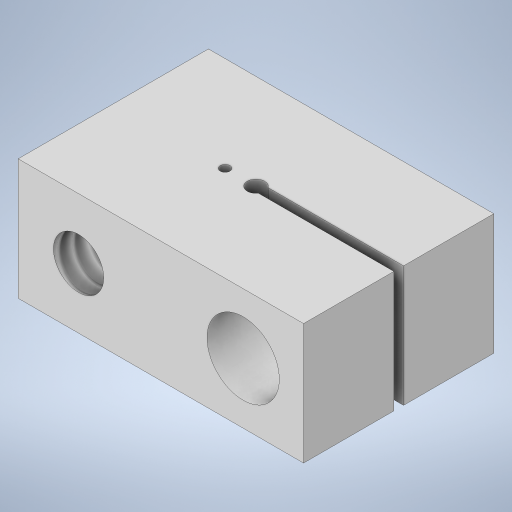
# Autodesk Inventor part: clamp(6-32)-th
Saved by Autodesk Inventor 2024 (Build 280153000, 153)
## iProperties
Created: 2023-04-27
Part Number: clamp(6-32)-th
Material: Generic
Document SubType Name: Modeling
Designer: Fujitsu
Density: 1 g/cm^3
Appearance: Default
Author: Fujitsu
Autodesk Inventor part; units mm, degrees
ref_plane "YZ Plane" through (0, 0, 0) normal (1, 0, 0) x (0, 1, 0)
ref_plane "XZ Plane" through (0, 0, 0) normal (0, 1, 0) x (-1, 0, 0)
ref_plane "XY Plane" through (0, 0, 0) normal (0, 0, 1) x (1, 0, 0)
sketch "Sketch1" plane through (0, 0, 0) normal (0, 1, 0) x (-1, 0, 0)
  line L0 (0, 0) -> (15, 0)
  line L1 (15, 0) -> (15, -10)
  line L2 (15, -10) -> (0, -10)
  line L3 (0, -10) -> (0, 0)
  line L4 (0, -5) -> (7.5006, -5)
  circle A0 centre (7.5006, -5) radius 0.4572
  line L5 (0, -5.254) -> (7.1205, -5.254)
  line L6 (0, -4.746) -> (7.1205, -4.746)
  dimension "d0" = 15
  dimension "d1" = 10
  dimension "d2" = 7.5006
  dimension "d3" = 0.9144
  dimension "d4" = 0.254
  dimension "d5" = 0.254
  constraints: 14 end point, 4 parallel, 2 horizontal, 2 point on circle, 1 centre point, 1 coincident, 1 midpoint, 1 perpendicular
  measures "d0" distance of L1.end L2.end
  measures "d1" distance of L0.end L1.end
  measures "d2" distance of L4.start L4.end
  measures "d3" diameter of A0
  measures "d4" distance between parallel lines of L4 L5
  measures "d5" distance between parallel lines of L4 L6
extrude "Extrusion1" add sketch "Sketch1" along normal blind 6.35 contours L0 L1 L2 L3 L5 A0 L6
sketch "Sketch2" plane through (-15, 0, 0) normal (0, 0, 1) x (1, 0, 0)
  line L0 (7.8795, 0) -> (15, 0) projected
  line L1 (15, 0) -> (8.65, 6.35)
  line L2 (15, 6.35) -> (7.8795, 6.35) projected
  line L3 (15, 0) -> (23.9803, 0) construction
  circle A0 centre (11.825, 3.175) radius 1.7526
  line L4 (15, 0) -> (0, 0) projected
  line L5 (0, 0) -> (6.35, 6.35)
  line L6 (7.0422, 6.35) -> (7.8795, 6.35) projected
  line L7 (0, 0) -> (8.9803, 0) construction
  circle A1 centre (3.175, 3.175) radius 1.7526
  dimension "d8" = 135
  dimension "d9" = 3.5052
  dimension "d10" = 45
  dimension "d11" = 3.5052
  constraints: 8 end point, 2 centre point, 2 equal length, 2 horizontal, 2 midpoint, 2 point on line
  measures "d8" angle of L3 L1
  measures "d9" diameter of A0
  measures "d10" angle of L7 L5
  measures "d11" diameter of A1
sketch "Sketch3" plane through (-15, 0, -10) normal (-1, 0, 0) x (0, 0, 1)
  line L0 (0, 6.35) -> (10, 6.35) projected
  line L1 (0, 6.35) -> (10, 0)
  circle A0 centre (5, 3.175) radius 0.508
  dimension "d30" = 1.016
  constraints: 2 end point, 1 centre point, 1 midpoint
  measures "d30" diameter of A0
extrude "Extrusion2" cut sketch "Sketch3" against normal blind 3.5001
hole "Hole3" at (-11.825, 3.175, 0) direction (0, 0, -1) diameter 2.6416 end through all thread size "6-32 UNC" class "2B" standard "ANSI Unified Screw Threads"
sketch "Sketch4" plane through (0, 0, -10) normal (0, 0, -1) x (-1, 0, 0)
  line L0 (0, 0) -> (6.35, 6.35)
  line L1 (7.1205, 6.35) -> (0, 6.35) projected
  line L2 (0, 0) -> (8.9803, 0) construction
  line L3 (6.35, 6.35) -> (3.175, 3.175)
  circle A0 centre (3.175, 3.175) radius 1.3208
  dimension "d44" = 45
  dimension "d45" = 2.6416
  constraints: 6 end point, 1 centre point, 1 coincident, 1 equal length, 1 horizontal, 1 midpoint, 1 point on line
  measures "d44" angle of L2 L0
  measures "d45" diameter of A0
hole "Hole4" at (-3.175, 3.175, -10) direction (0, 0, 1) diameter 2.6416 depth 5 tip angle 118 thread size "6-32 UNC" class "2B" standard "ANSI Unified Screw Threads"
hole "Hole5" at (-3.175, 3.175, 0) direction (0, 0, -1) diameter 3.7973 depth 5 tip angle 118 clearance for "Flat Head Machine Screw (82)" size "#6" standard "Ansi Unified Screw Threads"
sketch "Sketch5" plane through (0, 6.35, 0) normal (0, 1, 0) x (1, 0, 0)
  arc A0 (-7.1205, 5.254) -> (-7.1205, 4.746) centre (-7.5006, 5) ccw projected
  circle A1 centre (-7.5006, 5) radius 3.81
  circle A2 centre (-7.5006, 5) radius 16.51
  line L0 (-15, 10) -> (-15, 0) projected
  line L1 (-15, 0) -> (-8.65, 0)
  line L2 (-8.65, 0) -> (-8.65, -6.35)
  line L3 (-8.65, -6.35) -> (-15, -6.35)
  line L4 (-15, -6.35) -> (-15, 0)
  line L5 (-15, 10) -> (-8.65, 10)
  line L6 (-8.65, 10) -> (-8.65, 16.35)
  line L7 (-8.65, 16.35) -> (-15, 16.35)
  line L8 (-15, 16.35) -> (-15, 10)
  circle A3 centre (-7.5006, 5) radius 18.4277
  line L9 (-11.825, -9.8552) -> (-14.6952, -9.8552)
  line L10 (-14.6952, -9.8552) -> (-14.6952, -6.35)
  line L11 (-11.825, -9.8552) -> (-8.9548, -9.8552)
  line L12 (-8.9548, -9.8552) -> (-8.9548, -6.35)
  point P0 (0, 0)
  dimension "d60" = 7.62
  dimension "d61" = 33.02
  dimension "d62" = 6.35
  dimension "d63" = 6.35
  dimension "d64" = 6.35
  dimension "d65" = 6.35
  dimension "d66" = 36.8554
  dimension "d68" = 2.8702
  dimension "d69" = 2.8702
  constraints: 24 end point, 4 parallel, 4 perpendicular, 3 centre point, 3 coincident, 2 horizontal, 2 point on line, 1 vertical
  measures "d60" diameter of A1
  measures "d61" diameter of A2
  measures "d62" distance of L2.end L3.end
  measures "d63" distance of L1.end L2.end
  measures "d64" distance of L7.end L6.end
  measures "d65" distance of L6.end L5.end
  measures "d66" diameter of A3
  measures "d68" distance of L9.start L9.end
  measures "d69" distance of L9.start L11.end
sketch "Sketch6" plane through (0, 6.35, 0) normal (0, 1, 0) x (1, 0, 0)
  arc A0 (-7.1205, 5.254) -> (-7.1205, 4.746) centre (-7.5006, 5) ccw projected
  line L0 (-7.9578, 5) -> (-8.8722, 5)
  line L1 (-8.8722, 5) -> (-9.3802, 5)
  circle A1 centre (-9.1262, 5) radius 0.254
  point P0 (0, 0)
  dimension "d70" = 0.9144
  dimension "d71" = 0.508
  constraints: 4 end point, 1 horizontal, 1 horizontal alignment, 1 midpoint, 1 point on circle, 1 point on line, 2 other
  measures "d70" distance of L0.start L0.end
  measures "d71" distance of L0.end L1.end
hole "Hole6" at (-9.1262, 6.35, -5) direction (0, -1, 0) diameter 0.508 depth 0.508
body "Solid1"
